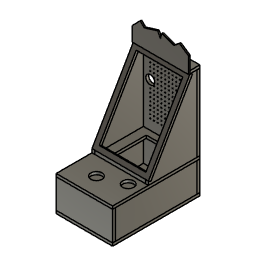
Decisioninator CAD Fusion 360 (Autodesk Fusion 360 design; units mm, degrees)
Autodesk Fusion 360 part; units mm, degrees
(part 1 of 2)
sketch "Front Bezel Sketch" plane through (0, 0, 0) normal (0, 1, 0) x (1, 0, 0)
  line L0 (-63, 93) -> (63, 93)
  line L1 (63, 93) -> (63, -93)
  line L2 (63, -93) -> (-63, -93)
  line L3 (-63, -93) -> (-63, 93)
  line L4 (-63, 93) -> (63, -93) construction
  line L5 (63, 93) -> (-63, -93) construction
  line L6 (50, 80) -> (-50, 80)
  line L7 (-50, 80) -> (-50, -80)
  line L8 (-50, -80) -> (50, -80)
  line L9 (50, -80) -> (50, 80)
  line L10 (50, 80) -> (-50, -80) construction
  line L11 (-50, 80) -> (50, -80) construction
  dimension "d3" = 126
  dimension "d4" = 186
  dimension "d5" = 100
  dimension "d6" = 160
  constraint horizontal L0
  constraint perpendicular L0 L1
  constraint parallel L0 L2
  constraint parallel L1 L3
  constraint coincident L4 origin
  constraint coincident L5 origin
  constraint horizontal L6
  constraint perpendicular L6 L7
  constraint parallel L6 L8
  constraint parallel L7 L9
  constraint coincident L10 origin
  constraint coincident L11 origin
  measures "d3" distance of L1.end L2.end
  measures "d4" distance of L0.end L1.end
  measures "d5" distance of L7.end L8.end
  measures "d6" distance of L6.end L7.end
extrude "Extrude1" add sketch "Front Bezel Sketch" along normal blind 6.35 makes body 1
sketch "Top Case Sketch" plane through (0, 6.35, 0) normal (0, 1, 0) x (-1, 0, 0)
  line L0 (-50, -80) -> (-50, 80)
  line L1 (-50, 80) -> (50, 80)
  line L2 (50, 80) -> (50, -80)
  line L3 (50, -80) -> (-50, -80)
  line L4 (63, 93) -> (-63, 93)
  line L5 (-63, 93) -> (-63, -93)
  line L6 (-63, -93) -> (63, -93)
  line L7 (63, -93) -> (63, 93)
  line L8 (-56.65, 86.65) -> (56.65, 86.65)
  line L9 (56.65, 86.65) -> (56.65, -86.65)
  line L10 (56.65, -86.65) -> (-56.65, -86.65)
  line L11 (-56.65, -86.65) -> (-56.65, 86.65)
  dimension "d9" = 6.35
  dimension "d10" = 6.35
  dimension "d11" = 6.35
  dimension "d12" = 6.35
  constraint horizontal L8
  constraint vertical L9
  constraint horizontal L10
  constraint vertical L11
  measures "d9" distance of L5 L11
  measures "d10" distance of L7 L9
  measures "d11" distance of L4 L8
  measures "d12" distance of L6 L10
move_body "Move1" bodies 1 to x (1, 0, 0) y (0, 0.866025, -0.5) z (0, 0.5, 0.866025) at (0, -42.6114, 14.8206)
sketch "Side" plane through (63, 0, 0) normal (1, 0, 0) x (0, 1, 0)
  line L0 (3.8886, 95.361) -> (-89.1114, -65.7197)
  line L1 (-89.1114, -65.7197) -> (-83.6122, -68.8947)
  line L2 (-83.6122, -68.8947) -> (9.3878, 92.186)
  line L3 (9.3878, 92.186) -> (3.8886, 95.361)
  line L4 (-83.6122, -68.8947) -> (10, -68.8947)
  line L5 (9.3878, 92.186) -> (9.3878, -70)
  constraint coincident L1.end L2.start
  constraint horizontal L4
  constraint coincident L2.end L3.start
  constraint perpendicular L4 L5
extrude "Extrude12" add sketch "Side" against normal blind 6.35 separate body contours L2 L4 L5 makes body 2
sketch "Sketch6" plane through (56.65, 0, 0) normal (-1, 0, 0) x (0, -1, 0)
  line L0 (-9.3878, -68.8947) -> (83.6122, -68.8947)
  line L1 (83.6122, -68.8947) -> (-9.3878, 92.186)
  line L2 (-9.3878, 92.186) -> (-9.3878, -68.8947)
extrude "Extrude13" add 1 faces at (60.8833, 9.3878, 38.4924) along direction (0, 1, 0) blind 10 on bodies 2 bodies 2
sketch "Sketch7" plane through (63, 0, 0) normal (1, 0, 0) x (0, 1, 0)
  line L0 (-83.6122, -68.8947) -> (19.3878, -68.8947)
  line L1 (19.3878, -68.8947) -> (19.3878, 92.186)
  line L2 (19.3878, 92.186) -> (9.3878, 92.186)
  line L3 (9.3878, 92.186) -> (-83.6122, -68.8947)
  line L4 (3.8886, 95.361) -> (9.3878, 92.186)
  line L5 (-89.1114, -65.7197) -> (3.8886, 95.361)
  line L6 (-83.6122, -68.8947) -> (9.3878, 92.186)
  line L7 (3.8886, 95.361) -> (20, 95.361)
  line L8 (19.3878, 92.186) -> (19.3878, 95.361)
  point P0 (3.8886, 95.361)
  point P1 (9.3878, 92.186)
  constraint coincident P0 L4.start
  constraint horizontal L7
  constraint coincident L1.end L2.start
  constraint coincident L7 L8.end
  constraint perpendicular L7 L8
extrude "Extrude14" add sketch "Sketch7" against normal blind 6.35 contours L2 L4 L7 L8 bodies 2
copy_body "CopyPasteBodies1" bodies 2 makes body 3
extrude "Extrude15" add 1 faces at (60.8833, -49.2788, -68.8947) along direction (0, 0, -1) blind 5 on bodies 2 bodies 2 3
sketch "Sketch8" plane through (63, 0, 0) normal (1, 0, 0) x (0, 1, 0)
  line L0 (3.8886, 95.361) -> (-89.1114, -65.7197)
  line L1 (-89.1114, -65.7197) -> (-83.6122, -68.8947)
  line L2 (-83.6122, -68.8947) -> (9.3878, 92.186)
  line L3 (9.3878, 92.186) -> (3.8886, 95.361)
  line L4 (-89.1114, -65.7197) -> (-89.1114, -73.8947)
  line L5 (-89.1114, -73.8947) -> (-83.5716, -73.8947)
  line L6 (-83.6122, -68.8947) -> (-83.6122, -73.8947)
  line L7 (19.3878, -73.8947) -> (-83.6122, -73.8947)
  constraint coincident L0.end L1.start
  constraint parallel L4 L6
  constraint collinear L5 L7
extrude "Extrude16" add sketch "Sketch8" against normal blind 6.35 contours L1 L4 L5 L6 bodies 2
copy_body "CopyPasteBodies2" bodies 2 makes body 4
move_body "Move3" bodies 4 to x (1, 0, 0) y (0, 1, 0) z (0, 0, 1) at (-110, 0, 0)
move_body "Align2" bodies 4 to x (1, 0, 0) y (0, 1, 0) z (0, 0, 1) at (-9.65, 0, 0)
sketch "Sketch9" plane through (56.65, 0, 0) normal (-1, 0, 0) x (0, -1, 0)
  line L0 (83.6122, -68.8947) -> (-9.3878, 92.186)
  line L1 (-9.3878, 92.186) -> (-3.8886, 95.361)
  line L2 (-3.8886, 95.361) -> (-19.3878, 95.361)
  line L3 (-19.3878, 95.361) -> (-19.3878, -73.8947)
  line L4 (-19.3878, -73.8947) -> (89.1114, -73.8947)
  line L5 (89.1114, -73.8947) -> (89.1114, -65.7197)
  line L6 (89.1114, -65.7197) -> (83.6122, -68.8947)
  line L7 (89.1114, -65.7197) -> (83.6122, -68.8947)
  line L8 (89.1114, -65.7197) -> (89.1114, -73.8947)
  line L9 (83.6122, -68.8947) -> (83.6122, -73.8947)
  line L10 (89.1114, -73.8947) -> (83.5716, -73.8947)
extrude "Extrude17" add sketch "Sketch9" along normal up to surface (113.3 mm away) separate body contours L4 L5 L6 L7 L8 L9 L10 makes body 5
sketch "Sketch10" plane through (0, 19.3878, 0) normal (0, 1, 0) x (-1, 0, 0)
  line L0 (-63, 95.361) -> (-63, -73.8947)
  line L1 (-63, -73.8947) -> (-56.65, -73.8947)
  line L2 (-56.65, -73.8947) -> (-56.65, 95.361)
  line L3 (-56.65, 95.361) -> (-63, 95.361)
  line L4 (63, 95.361) -> (63, -73.8947)
  line L5 (-56.65, -73.8947) -> (56.65, -73.8947)
  line L6 (63, -73.8947) -> (56.65, -73.8947)
  line L7 (-56.65, -73.8947) -> (-63, -73.8947)
  line L8 (-63, -68.8947) -> (-63, 92.186)
  line L9 (-63, 92.186) -> (-63, 95.361)
  line L10 (-63, 95.361) -> (-56.65, 95.361)
  line L11 (-63, 95.361) -> (63, 95.361)
  line L12 (-63, 95.361) -> (63, 95.361)
  line L13 (63, 95.361) -> (63, -73.8947)
  line L14 (63, -73.8947) -> (-63, -73.8947)
  line L15 (-63, -73.8947) -> (-63, 95.361)
  point P0 (63, -73.8947)
  constraint horizontal L12
  constraint vertical L13
  constraint horizontal L14
  constraint vertical L15
  constraint coincident P0 L4.end
  constraint coincident L0.start L3.end
extrude "Extrude18" add sketch "Sketch10" along normal blind 6.35 separate body makes body 6
sketch "Sketch11" plane through (0, 25.7378, 0) normal (0, 1, 0) x (-1, 0, 0)
  line L0 (-63, -73.8947) -> (63, -73.8947)
  line L1 (63, -73.8947) -> (63, 95.361)
  line L2 (63, 95.361) -> (-63, 95.361)
  line L3 (-63, 95.361) -> (-63, -73.8947)
  line L4 (-46.65, 79.011) -> (46.65, 79.011)
  line L5 (46.65, 79.011) -> (46.65, -57.5447)
  line L6 (46.65, -57.5447) -> (-46.65, -57.5447)
  line L7 (-46.65, -57.5447) -> (-46.65, 79.011)
  circle A0 centre (-41.65, 74.011) radius 1.25
  dimension "d63" = 16.35
  dimension "d64" = 16.35
  dimension "d65" = 16.35
  dimension "d66" = 16.35
  dimension "d67" = 2.5
  dimension "d68" = 5
  dimension "d69" = 5
  constraint horizontal L4
  constraint vertical L5
  constraint horizontal L6
  constraint vertical L7
  measures "d63" distance of L3 L7
  measures "d64" distance of L1 L5
  measures "d65" distance of L2 L4
  measures "d66" distance of L0 L6
  measures "d67" diameter of A0
  measures "d68" distance of L7 A0.centre
  measures "d69" distance of L4 A0.centre
extrude "Extrude19" cut sketch "Sketch11" against normal blind 6.35 contours A0 bodies 6
pattern_linear "R-Pattern4" count 16 spacing 8.3333 along (0, 0, -1) count 11 spacing 8.3 along (-1, 0, 0) of "Extrude19"
extrude "Extrude20" add 1 faces at (58.7667, 9.055, 95.361) along direction (0, 0, 1) blind 6.35 separate body on bodies 2 makes body 7
extrude "Extrude21" add 1 faces at (-60.8833, 9.055, 95.361) along direction (0, 0, 1) blind 6.35 separate body on bodies 4 makes body 8
extrude "Extrude22" add 1 faces at (-56.65, 9.055, 97.4777) along direction (1, 0, 0) up to near side of body 7 separate body on bodies 8 makes body 9
combine "Combine1" operation add target body 9 tool bodies 8
combine "Combine2" operation add target body 9 tool bodies 7
extrude "Extrude23" add 1 faces at (60.8833, -52.945, -73.8947) along direction (0, 0, -1) blind 6.35 separate body on bodies 2 makes body 10
extrude "Extrude24" add 1 faces at (60.8833, 19.3878, -76.0114) along direction (0, 1, 0) blind 6.35 on bodies 10 bodies 10
extrude "Extrude25" add 1 faces at (56.65, -12.5452, -76.0114) along direction (-1, 0, 0) blind 119.65 on bodies 10 bodies 10
extrude "Extrude26" add 1 faces at (-21, -89.1114, -78.128) along direction (0, -1, 0) blind 80 on bodies 10 bodies 10
sketch "Sketch12" plane through (0, 0, -73.8947) normal (0, 0, 1) x (-1, 0, 0)
  line L0 (-63, 169.1114) -> (-63, -25.7378)
  line L1 (-63, -25.7378) -> (63, -25.7378)
  line L2 (63, -25.7378) -> (63, 169.1114)
  line L3 (63, 169.1114) -> (-63, 169.1114)
  line L4 (36.65, -5.7378) -> (-36.65, -5.7378)
  line L5 (-36.65, -5.7378) -> (-36.65, 69.1114)
  line L6 (-36.65, 69.1114) -> (36.65, 69.1114)
  line L7 (36.65, 69.1114) -> (36.65, -5.7378)
  line L8 (56.65, -19.3878) -> (56.65, 89.1114)
  line L9 (-56.65, -19.3878) -> (-56.65, 89.1114)
  dimension "d90" = 20
  dimension "d91" = 20
  dimension "d92" = 20
  dimension "d93" = 20
  constraint horizontal L4
  constraint vertical L5
  constraint horizontal L6
  constraint vertical L7
  measures "d90" distance of L7 L8
  measures "d91" distance of L5 L9
  measures "d92" distance of L1 L4
  measures "d93" distance of L6 L8.end
extrude "Extrude27" cut sketch "Sketch12" against normal blind 6.35 contours L4 L5 L6 L7 bodies 10
extrude "Extrude28" add 1 faces at (21, 19.3878, 99.5943) along direction (0, 1, 0) blind 6.35 on bodies 9 bodies 9
sketch "Sketch13" plane through (0, 0, -80.2447) normal (0, 0, -1) x (1, 0, 0)
  line L0 (36.65, 69.1114) -> (36.65, -5.7378)
  line L1 (36.65, -5.7378) -> (-36.65, -5.7378)
  line L2 (-36.65, -5.7378) -> (-36.65, 69.1114)
  line L3 (-36.65, 69.1114) -> (36.65, 69.1114)
  line L4 (63, -25.7378) -> (63, 169.1114)
  line L5 (63, 169.1114) -> (-63, 169.1114)
  line L6 (-63, 169.1114) -> (-63, -25.7378)
  line L7 (-63, -25.7378) -> (63, -25.7378)
  line L8 (-63, 162.7614) -> (63, 162.7614)
  line L9 (-63, -19.3878) -> (63, -19.3878)
  line L10 (56.65, 162.7614) -> (56.65, -19.3878)
  line L11 (-56.65, 162.7614) -> (-56.65, -19.3878)
  dimension "d98" = 6.35
  dimension "d99" = 6.35
  dimension "d100" = 6.35
  dimension "d101" = 6.35
  constraint coincident L6 L8.start
  constraint coincident L4 L8.end
  constraint perpendicular L4 L8
  constraint coincident L6 L9.start
  constraint coincident L4 L9.end
  constraint perpendicular L4 L9
  constraint coincident L8 L10.start
  constraint coincident L9 L10.end
  constraint perpendicular L9 L10
  constraint coincident L8 L11.start
  constraint perpendicular L1 L11
  measures "d98" distance of L5 L8
  measures "d99" distance of L7 L9
  measures "d100" distance of L6 L11
  measures "d101" distance of L4 L10
extrude "Extrude29" add sketch "Sketch13" along normal blind 80 separate body contours L4 L5 L6 L8 makes body 11
extrude "Extrude30" add sketch "Sketch13" along normal blind 80 separate body contours L6 L8 L9 L11 makes body 12
extrude "Extrude31" add sketch "Sketch13" along normal blind 80 separate body contours L4 L6 L7 L9 makes body 13
extrude "Extrude32" add sketch "Sketch13" along normal blind 80 separate body contours L4 L8 L9 L10 makes body 14
extrude "Extrude33" cut 4 faces at (60.8833, -41.3286, -160.2447) (18.8833, 23.6212, -160.2447) (-58.7667, -102.045, -160.2447) (-18.8833, -166.9948, -160.2447) along direction (0, 0, 1) blind 15 on bodies 11 12 13 14 bodies 11 12 13 14
sketch "Sketch14" plane through (0, 0, -145.2447) normal (0, 0, -1) x (1, 0, 0)
  line L0 (63, -19.3878) -> (-63, -19.3878)
  line L1 (-63, -19.3878) -> (-63, -25.7378)
  line L2 (-63, -25.7378) -> (63, -25.7378)
  line L3 (63, -25.7378) -> (63, -19.3878)
  line L4 (63, -25.7378) -> (-63, -25.7378)
  line L5 (-63, -25.7378) -> (-63, 169.1114)
  line L6 (-63, 169.1114) -> (63, 169.1114)
  line L7 (63, 169.1114) -> (63, -25.7378)
  line L8 (-63, 169.1114) -> (-63, -25.7378)
  line L9 (63, 169.1114) -> (-63, 169.1114)
  constraint horizontal L4
  constraint vertical L5
  constraint horizontal L6
  constraint vertical L7
  constraint coincident L2.end L3.start
  constraint collinear L5 L8
  constraint collinear L6 L9
extrude "Extrude34" add sketch "Sketch14" along normal blind 6.35 separate body makes body 15
sketch "Sketch15" plane through (0, 25.7378, 0) normal (0, 1, 0) x (-1, 0, 0)
  circle A0 centre (41.35, -50.989) radius 1.25
  circle A1 centre (41.35, -42.6557) radius 1.25
  circle A2 centre (41.35, -34.3223) radius 1.25
  circle A3 centre (41.35, -25.989) radius 1.25
  circle A4 centre (41.35, -17.6557) radius 1.25
  circle A5 centre (41.35, -9.3223) radius 1.25
  circle A6 centre (41.35, -0.989) radius 1.25
  circle A7 centre (41.35, 7.3443) radius 1.25
  circle A8 centre (41.35, 15.6777) radius 1.25
  circle A9 centre (41.35, 24.011) radius 1.25
  circle A10 centre (41.35, 32.3443) radius 1.25
  circle A11 centre (41.35, 40.6777) radius 1.25
  circle A12 centre (41.35, 49.011) radius 1.25
  circle A13 centre (41.35, 57.3443) radius 1.25
  circle A14 centre (41.35, 65.6777) radius 1.25
  circle A15 centre (41.35, 74.011) radius 1.25
  circle A16 centre (33.05, -50.989) radius 1.25
  circle A17 centre (33.05, -42.6557) radius 1.25
  circle A18 centre (33.05, -34.3223) radius 1.25
  circle A19 centre (33.05, -25.989) radius 1.25
  circle A20 centre (33.05, -17.6557) radius 1.25
  circle A21 centre (33.05, -9.3223) radius 1.25
  circle A22 centre (33.05, -0.989) radius 1.25
  circle A23 centre (33.05, 7.3443) radius 1.25
  circle A24 centre (33.05, 15.6777) radius 1.25
  circle A25 centre (33.05, 24.011) radius 1.25
  circle A26 centre (33.05, 32.3443) radius 1.25
  circle A27 centre (33.05, 40.6777) radius 1.25
  circle A28 centre (33.05, 49.011) radius 1.25
  circle A29 centre (33.05, 57.3443) radius 1.25
  circle A30 centre (33.05, 65.6777) radius 1.25
  circle A31 centre (33.05, 74.011) radius 1.25
  circle A32 centre (24.75, -50.989) radius 1.25
  circle A33 centre (24.75, -42.6557) radius 1.25
  circle A34 centre (24.75, -34.3223) radius 1.25
  circle A35 centre (24.75, -25.989) radius 1.25
  circle A36 centre (24.75, -17.6557) radius 1.25
  circle A37 centre (24.75, -9.3223) radius 1.25
  circle A38 centre (24.75, -0.989) radius 1.25
  circle A39 centre (24.75, 7.3443) radius 1.25
  circle A40 centre (24.75, 15.6777) radius 1.25
  circle A41 centre (24.75, 24.011) radius 1.25
  circle A42 centre (24.75, 32.3443) radius 1.25
  circle A43 centre (24.75, 40.6777) radius 1.25
  circle A44 centre (24.75, 49.011) radius 1.25
  circle A45 centre (24.75, 57.3443) radius 1.25
  circle A46 centre (24.75, 65.6777) radius 1.25
  circle A47 centre (24.75, 74.011) radius 1.25
  circle A48 centre (16.45, -50.989) radius 1.25
  circle A49 centre (16.45, -42.6557) radius 1.25
  circle A50 centre (16.45, -34.3223) radius 1.25
  circle A51 centre (16.45, -25.989) radius 1.25
  circle A52 centre (16.45, -17.6557) radius 1.25
  circle A53 centre (16.45, -9.3223) radius 1.25
  circle A54 centre (16.45, -0.989) radius 1.25
  circle A55 centre (16.45, 7.3443) radius 1.25
  circle A56 centre (16.45, 15.6777) radius 1.25
  circle A57 centre (16.45, 24.011) radius 1.25
  circle A58 centre (16.45, 32.3443) radius 1.25
  circle A59 centre (16.45, 40.6777) radius 1.25
  circle A60 centre (16.45, 49.011) radius 1.25
  circle A61 centre (16.45, 57.3443) radius 1.25
  circle A62 centre (16.45, 65.6777) radius 1.25
  circle A63 centre (16.45, 74.011) radius 1.25
  circle A64 centre (8.15, -50.989) radius 1.25
  circle A65 centre (8.15, -42.6557) radius 1.25
  circle A66 centre (8.15, -34.3223) radius 1.25
  circle A67 centre (8.15, -25.989) radius 1.25
  circle A68 centre (8.15, -17.6557) radius 1.25
  circle A69 centre (8.15, -9.3223) radius 1.25
  circle A70 centre (8.15, -0.989) radius 1.25
  circle A71 centre (8.15, 7.3443) radius 1.25
  circle A72 centre (8.15, 15.6777) radius 1.25
  circle A73 centre (8.15, 24.011) radius 1.25
  circle A74 centre (8.15, 32.3443) radius 1.25
  circle A75 centre (8.15, 40.6777) radius 1.25
  circle A76 centre (8.15, 49.011) radius 1.25
  circle A77 centre (8.15, 57.3443) radius 1.25
  circle A78 centre (8.15, 65.6777) radius 1.25
  circle A79 centre (8.15, 74.011) radius 1.25
  circle A80 centre (-0.15, -50.989) radius 1.25
  circle A81 centre (-0.15, -42.6557) radius 1.25
  circle A82 centre (-0.15, -34.3223) radius 1.25
  circle A83 centre (-0.15, -25.989) radius 1.25
  circle A84 centre (-0.15, -17.6557) radius 1.25
  circle A85 centre (-0.15, -9.3223) radius 1.25
  circle A86 centre (-0.15, -0.989) radius 1.25
  circle A87 centre (-0.15, 7.3443) radius 1.25
  circle A88 centre (-0.15, 15.6777) radius 1.25
  circle A89 centre (-0.15, 24.011) radius 1.25
  circle A90 centre (-0.15, 32.3443) radius 1.25
  circle A91 centre (-0.15, 40.6777) radius 1.25
  circle A92 centre (-0.15, 49.011) radius 1.25
  circle A93 centre (-0.15, 57.3443) radius 1.25
  circle A94 centre (-0.15, 65.6777) radius 1.25
  circle A95 centre (-0.15, 74.011) radius 1.25
  circle A96 centre (-8.45, -50.989) radius 1.25
  circle A97 centre (-8.45, -42.6557) radius 1.25
  circle A98 centre (-8.45, -34.3223) radius 1.25
  circle A99 centre (-8.45, -25.989) radius 1.25
  circle A100 centre (-8.45, -17.6557) radius 1.25
  circle A101 centre (-8.45, -9.3223) radius 1.25
  circle A102 centre (-8.45, -0.989) radius 1.25
  circle A103 centre (-8.45, 7.3443) radius 1.25
  circle A104 centre (-8.45, 15.6777) radius 1.25
  circle A105 centre (-8.45, 24.011) radius 1.25
  circle A106 centre (-8.45, 32.3443) radius 1.25
  circle A107 centre (-8.45, 40.6777) radius 1.25
  circle A108 centre (-8.45, 49.011) radius 1.25
  circle A109 centre (-8.45, 57.3443) radius 1.25
  circle A110 centre (-8.45, 65.6777) radius 1.25
  circle A111 centre (-8.45, 74.011) radius 1.25
  circle A112 centre (-16.75, -50.989) radius 1.25
  circle A113 centre (-16.75, -42.6557) radius 1.25
  circle A114 centre (-16.75, -34.3223) radius 1.25
  circle A115 centre (-16.75, -25.989) radius 1.25
  circle A116 centre (-16.75, -17.6557) radius 1.25
  circle A117 centre (-16.75, -9.3223) radius 1.25
  circle A118 centre (-16.75, -0.989) radius 1.25
  circle A119 centre (-16.75, 7.3443) radius 1.25
  circle A120 centre (-16.75, 15.6777) radius 1.25
  circle A121 centre (-16.75, 24.011) radius 1.25
  circle A122 centre (-16.75, 32.3443) radius 1.25
  circle A123 centre (-16.75, 40.6777) radius 1.25
  circle A124 centre (-16.75, 49.011) radius 1.25
  circle A125 centre (-16.75, 57.3443) radius 1.25
  circle A126 centre (-16.75, 65.6777) radius 1.25
  circle A127 centre (-16.75, 74.011) radius 1.25
  circle A128 centre (-25.05, -50.989) radius 1.25
  circle A129 centre (-25.05, -42.6557) radius 1.25
  circle A130 centre (-25.05, -34.3223) radius 1.25
  circle A131 centre (-25.05, -25.989) radius 1.25
  circle A132 centre (-25.05, -17.6557) radius 1.25
  circle A133 centre (-25.05, -9.3223) radius 1.25
  circle A134 centre (-25.05, -0.989) radius 1.25
  circle A135 centre (-25.05, 7.3443) radius 1.25
  circle A136 centre (-25.05, 15.6777) radius 1.25
  circle A137 centre (-25.05, 24.011) radius 1.25
  circle A138 centre (-25.05, 32.3443) radius 1.25
  circle A139 centre (-25.05, 40.6777) radius 1.25
  circle A140 centre (-25.05, 49.011) radius 1.25
  circle A141 centre (-25.05, 57.3443) radius 1.25
  circle A142 centre (-25.05, 65.6777) radius 1.25
  circle A143 centre (-25.05, 74.011) radius 1.25
  circle A144 centre (-33.35, -50.989) radius 1.25
  circle A145 centre (-33.35, -42.6557) radius 1.25
  circle A146 centre (-33.35, -34.3223) radius 1.25
  circle A147 centre (-33.35, -25.989) radius 1.25
  circle A148 centre (-33.35, -17.6557) radius 1.25
  circle A149 centre (-33.35, -9.3223) radius 1.25
  circle A150 centre (-33.35, -0.989) radius 1.25
  circle A151 centre (-33.35, 7.3443) radius 1.25
  circle A152 centre (-33.35, 15.6777) radius 1.25
  circle A153 centre (-33.35, 24.011) radius 1.25
  circle A154 centre (-33.35, 32.3443) radius 1.25
  circle A155 centre (-33.35, 40.6777) radius 1.25
  circle A156 centre (-33.35, 49.011) radius 1.25
  circle A157 centre (-33.35, 57.3443) radius 1.25
  circle A158 centre (-33.35, 65.6777) radius 1.25
  circle A159 centre (-33.35, 74.011) radius 1.25
  circle A160 centre (-41.65, -50.989) radius 1.25
  circle A161 centre (-41.65, -42.6557) radius 1.25
  circle A162 centre (-41.65, -34.3223) radius 1.25
  circle A163 centre (-41.65, -25.989) radius 1.25
  circle A164 centre (-41.65, -17.6557) radius 1.25
  circle A165 centre (-41.65, -9.3223) radius 1.25
  circle A166 centre (-41.65, -0.989) radius 1.25
  circle A167 centre (-41.65, 7.3443) radius 1.25
  circle A168 centre (-41.65, 15.6777) radius 1.25
  circle A169 centre (-41.65, 24.011) radius 1.25
  circle A170 centre (-41.65, 32.3443) radius 1.25
  circle A171 centre (-41.65, 40.6777) radius 1.25
  circle A172 centre (-41.65, 49.011) radius 1.25
  circle A173 centre (-41.65, 57.3443) radius 1.25
  circle A174 centre (-41.65, 65.6777) radius 1.25
  circle A175 centre (-41.65, 74.011) radius 1.25
  line L0 (-63, -73.8947) -> (63, -73.8947)
  line L1 (63, -73.8947) -> (63, 95.361)
  line L2 (63, 95.361) -> (-63, 95.361)
  line L3 (-63, 95.361) -> (-63, -73.8947)
  circle A176 centre (41.35, 24.011) radius 10
  dimension "d114" = 20
  constraint coincident A9.centre A176.centre
  measures "d114" diameter of A176
extrude "Extrude35" cut sketch "Sketch15" against normal blind 20 contours A176 bodies 6
sketch "Sketch16" plane through (0, 0, -151.5947) normal (0, 0, -1) x (1, 0, 0)
  line L0 (63, -25.7378) -> (63, 169.1114)
  line L1 (63, 169.1114) -> (-63, 169.1114)
  line L2 (-63, 169.1114) -> (-63, -25.7378)
  line L3 (-63, -25.7378) -> (63, -25.7378)
  circle A0 centre (0, 0) radius 10
  dimension "d117" = 20
  constraint coincident A0.centre origin
  measures "d117" diameter of A0
extrude "Extrude36" cut sketch "Sketch16" against normal blind 50 contours A0 bodies 15
sketch "Sketch17" plane through (0, 0, -73.8947) normal (0, 0, 1) x (-1, 0, 0)
  line L0 (-36.65, -5.7378) -> (-36.65, 69.1114)
  line L1 (-36.65, 69.1114) -> (36.65, 69.1114)
  line L2 (36.65, 69.1114) -> (36.65, -5.7378)
  line L3 (36.65, -5.7378) -> (-36.65, -5.7378)
  line L4 (-63, 169.1114) -> (-63, -25.7378)
  line L5 (-63, -25.7378) -> (63, -25.7378)
  line L6 (63, -25.7378) -> (63, 169.1114)
  line L7 (63, 169.1114) -> (-63, 169.1114)
  circle A0 centre (13, 129.1114) radius 12.5
  circle A1 centre (13, 129.1114) radius 30.25
  circle A2 centre (-38, 109.1114) radius 16.5
  line L8 (-56.65, 89.1114) -> (56.65, 89.1114)
  circle A3 centre (-38, 109.1114) radius 12.5
  dimension "d120" = 25
  dimension "d121" = 50
  dimension "d122" = 40
  dimension "d124" = 60.5
  dimension "d125" = 33
  dimension "d126" = 20
  dimension "d127" = 25
  dimension "d128" = 25
  constraint concentric A0 A1
  constraint concentric A2 A3
  measures "d120" diameter of A0
  measures "d121" distance of L6 A0.centre
  measures "d122" distance of L7 A0.centre
  measures "d124" diameter of A1
  measures "d125" diameter of A2
  measures "d126" distance of A2.centre L8
  measures "d127" distance of L4 A2.centre
  measures "d128" diameter of A3
extrude "Extrude37" cut sketch "Sketch17" against normal blind 7.62 contours A0 bodies 10
extrude "Extrude38" cut sketch "Sketch17" against normal blind 7.62 contours A3 bodies 10
sketch "Sketch18" plane through (0, 0, 101.711) normal (0, 0, 1) x (-1, 0, 0)
  line L0 (63, -25.7378) -> (63, -3.8886)
  line L1 (63, -3.8886) -> (-63, -3.8886)
  line L2 (-63, -3.8886) -> (-63, -25.7378)
  line L3 (-63, -25.7378) -> (63, -25.7378)
  line L4 (63, -3.8886) -> (-63, -3.8886)
  line L5 (-63, -3.8886) -> (-63, -7.0636)
  line L6 (-63, -7.0636) -> (63, -7.0636)
  line L7 (63, -7.0636) -> (63, -3.8886)
  dimension "d133" = 3.175
  constraint horizontal L4
  constraint vertical L5
  constraint horizontal L6
  constraint vertical L7
  constraint coincident L2 L5.end
  constraint coincident L0.end L1.start
  measures "d133" distance of L4 L6
extrude "Extrude39" add sketch "Sketch18" along normal blind 50 separate body contours L0 L1 L2 L4 L5 L6 L7 makes body 16
sketch "Sketch19" plane through (0, 3.8886, 0) normal (0, -1, 0) x (1, 0, 0)
  line L0 (-63, 101.711) -> (63, 101.711)
  line L1 (63, 101.711) -> (63, 151.711)
  line L2 (63, 151.711) -> (-63, 151.711)
  line L3 (-63, 151.711) -> (-63, 101.711)
  line L4 (-63, 133.5614) -> (-45.2775, 151.711)
  line L5 (-45.2775, 151.711) -> (-35.984, 142.6362)
  line L6 (-35.984, 142.6362) -> (-6.8129, 151.711)
  line L7 (-5.8194, 151.711) -> (0, 140)
  line L8 (0, 140) -> (3.4065, 151.711)
  line L9 (3.4065, 151.711) -> (30.0903, 141.6517)
  line L10 (30.0903, 141.6517) -> (42.5807, 151.711)
  line L11 (42.5807, 151.711) -> (63, 137.9614)
  constraint coincident L3 L4.start
  constraint coincident L2 L4.end
  constraint perpendicular L4 L5
  constraint coincident L2 L6.end
  constraint coincident L2 L7.start
  constraint coincident L2 L8.end
  constraint coincident L2 L10.end
  constraint coincident L1 L11.end
extrude "Extrude40" cut sketch "Sketch19" against normal blind 85 contours L2 L3 L4 | L1 L2 L11 | L2 L5 L6 | L2 L9 L10 | L2 L7 L8 bodies 16
move_body "Align3" bodies 16 to x (1, 0, 0) y (0, 1, 0) z (0, 0, 1) at (0, -3.175, -6.35)
copy_body "CopyPasteBodies3" bodies 1 makes body 17
sketch "Sketch21" plane through (63, 0, 0) normal (1, 0, 0) x (0, 1, 0)
  line L0 (19.3878, -73.8947) -> (19.3878, 95.361)
  line L1 (19.3878, 95.361) -> (3.8886, 95.361)
  line L2 (3.8886, 95.361) -> (9.3878, 92.186)
  line L3 (9.3878, 92.186) -> (-83.6122, -68.8947)
  line L4 (-83.6122, -68.8947) -> (-89.1114, -65.7197)
  line L5 (-89.1114, -65.7197) -> (-89.1114, -73.8947)
  line L6 (-89.1114, -73.8947) -> (19.3878, -73.8947)
  line L7 (3.8886, 95.361) -> (-89.1114, -65.7197)
  line L8 (3.8886, 95.361) -> (3.8886, 101.711)
  line L9 (3.8886, 101.711) -> (25.7378, 101.711)
  line L10 (25.7378, 101.711) -> (25.7378, 95.361)
  line L11 (25.7378, 95.361) -> (25.7378, -73.8947)
  line L12 (25.7378, -73.8947) -> (25.7378, -80.2447)
  line L13 (25.7378, -80.2447) -> (25.7378, -145.2447)
  line L14 (25.7378, -145.2447) -> (25.7378, -151.5947)
  line L15 (25.7378, -151.5947) -> (-169.1114, -151.5947)
  line L16 (-169.1114, -145.2447) -> (-169.1114, -151.5947)
  line L17 (-169.1114, -80.2447) -> (-169.1114, -145.2447)
  line L18 (-169.1114, -80.2447) -> (-169.1114, -73.8947)
  line L19 (-89.1114, -65.7197) -> (-89.1114, -73.8947)
  line L20 (-169.1114, -73.8947) -> (-89.1114, -73.8947)
  constraint coincident L18.end L20.start
  constraint coincident L5.end L6.start
sketch "Sketch22" plane through (0, 0, -73.8947) normal (0, 0, 1) x (-1, 0, 0)
  circle A0 centre (-38, 109.1114) radius 12.5
  circle A1 centre (13, 129.1114) radius 12.5
  line L0 (-36.65, -5.7378) -> (-36.65, 69.1114)
  line L1 (-36.65, 69.1114) -> (36.65, 69.1114)
  line L2 (36.65, 69.1114) -> (36.65, -5.7378)
  line L3 (36.65, -5.7378) -> (-36.65, -5.7378)
  line L4 (-63, 169.1114) -> (-63, -25.7378)
  line L5 (-63, -25.7378) -> (63, -25.7378)
  line L6 (63, -25.7378) -> (63, 169.1114)
  line L7 (63, 169.1114) -> (-63, 169.1114)
  line L8 (63, 89.1114) -> (-63, 89.1114)
  line L9 (-63, 169.1114) -> (63, 169.1114)
  circle A2 centre (13, 129.1114) radius 12.5
  circle A3 centre (-38, 109.1114) radius 12.5
  line L10 (63, 89.1114) -> (63, 169.1114)
  line L11 (-63, 89.1114) -> (-63, 169.1114)
  constraint coincident L8.start L10.start
  constraint coincident L6.end L7.start
  constraint coincident L8.end L11.start
  constraint coincident L4.start L7.end
copy_body "CopyPasteBodies4" bodies 16 makes body 18
move_body "Move5" bodies 18 to x (1, 0, 0) y (0, 1, 0) z (0, 0, 1) at (230, 0, 0)
move_body "Align5" bodies 18 to x (1, 0, 0) y (0, 0, 1) z (0, -1, 0) at (0, 99.2496, -3.8886)
copy_body "CopyPasteBodies5" bodies 9 makes body 19
move_body "Move6" bodies 19 to x (1, 0, 0) y (0, 1, 0) z (0, 0, 1) at (600, 0, 0)
move_body "Align6" bodies 19 to x (1, 0, 0) y (0, -1, 0) z (0, 0, -1) at (0, 29.6264, 95.361)
move_body "Move7" bodies 19 to x (1, 0, 0) y (0, 1, 0) z (0, 0, 1) at (-370, 10, 0)
copy_body "CopyPasteBodies6" bodies 6 makes body 20
move_body "Move8" bodies 20 to x (1, 0, 0) y (0, 1, 0) z (0, 0, 1) at (410, 0, 0)
move_body "Align7" bodies 20 to x (1, 0, 0) y (0, 0, 1) z (0, -1, 0) at (0, 36.471, -25.7378)
move_body "Move9" bodies 20 to x (1, 0, 0) y (0, 1, 0) z (0, 0, 1) at (-40, -70, 0)
copy_body "CopyPasteBodies7" bodies 2 makes body 21
move_body "Move10" bodies 21 to x (1, 0, 0) y (0, 1, 0) z (0, 0, 1) at (440, 0, 0)
move_body "Align8" bodies 21 to x (0, 0, -1) y (0, 1, 0) z (1, 0, 0) at (485.0044, 0, 496.65)
move_body "Move11" bodies 21 to x (0, 1, 0) y (-1, 0, 0) z (0, 0, 1) at (465.1253, -536.3497, 0)
copy_body "CopyPasteBodies8" bodies 4 makes body 22
move_body "Move12" bodies 22 to x (1, 0, 0) y (0, 1, 0) z (0, 0, 1) at (760, 0, 0)
move_body "Align9" bodies 22 to x (0, 0, -1) y (0, 1, 0) z (1, 0, 0) at (685.3544, 0, 697)
move_body "Move13" bodies 22 to x (0, -1, 0) y (1, 0, 0) z (0, 0, 1) at (561.5285, 655.7115, 0)
move_body "Align10" bodies 22 to x (1, 0, 0) y (0, -1, 0) z (0, 0, -1) at (0, -82.5771, -6.35)
move_body "Move14" bodies 22 to x (-0.996195, -0.087156, 0) y (0.087156, -0.996195, 0) z (0, 0, 1) at (1029.922, -13.5464, -320)
move_body "Align11" bodies 22 to x (1, 0, 0) y (0, -1, 0) z (0, 0, -1) at (0, -36.2417, -326.35)
move_body "Move15" bodies 22 to x (0.996195, 0.087156, 0) y (-0.087156, 0.996195, 0) z (0, 0, 1) at (3.0201, -42.5908, 0)
move_body "Move16" bodies 22 to x (-1, 0, 0) y (0, -1, 0) z (0, 0, 1) at (1027.4435, -58.1734, 0)
copy_body "CopyPasteBodies9" bodies 17 makes body 23
move_body "Move17" bodies 23 to x (1, 0, 0) y (0, 1, 0) z (0, 0, 1) at (230, 0, 0)
move_body "Align12" bodies 23 to x (1, 0, 0) y (0, -0.5, 0.866025) z (0, -0.866025, -0.5) at (0, -45.5828, 37.9629)
move_body "Move18" bodies 23 to x (1, 0, 0) y (0, 1, 0) z (0, 0, 1) at (0, -10, 0)
move_body "Move19" bodies 18 to x (1, 0, 0) y (0, 1, 0) z (0, 0, 1) at (0, -200, 0)
move_body "Move20" bodies 19 to x (0, -1, 0) y (1, 0, 0) z (0, 0, 1) at (174.2622, 185.7378, 0)
move_body "Move21" bodies 18 to x (0, 1, 0) y (-1, 0, 0) z (0, 0, 1) at (28.6169, -270.8398, 0)
copy_body "CopyPasteBodies10" bodies 10 makes body 24
move_body "Move22" bodies 24 to x (1, 0, 0) y (0, 1, 0) z (0, 0, 1) at (190, -130, 0)
move_body "Align13" bodies 24 to x (1, 0, 0) y (0, -1, 0) z (0, 0, -1) at (0, -241.2243, -80.2447)
move_body "Move23" bodies 24 to x (1, 0, 0) y (0, 1, 0) z (0, 0, 1) at (40, -210, 0)
copy_body "CopyPasteBodies11" bodies 15 makes body 25
move_body "Move24" bodies 25 to x (1, 0, 0) y (0, 1, 0) z (0, 0, 1) at (290, 0, 0)
move_body "Align14" bodies 25 to x (1, 0, 0) y (0, -1, 0) z (0, 0, -1) at (0, -143.3736, -151.5947)
move_body "Move25" bodies 25 to x (1, 0, 0) y (0, 1, 0) z (0, 0, 1) at (80, -170, 0)
copy_body "CopyPasteBodies12" bodies 11 makes body 26
move_body "Move26" bodies 26 to x (1, 0, 0) y (0, 1, 0) z (0, 0, 1) at (500, 0, 0)
move_body "Align15" bodies 26 to x (1, 0, 0) y (0, 0, 1) z (0, -1, 0) at (0, -243.0061, 162.7614)
move_body "Move27" bodies 26 to x (1, 0, 0) y (0, 1, 0) z (0, 0, 1) at (10, -40, 0)
copy_body "CopyPasteBodies13" bodies 13 makes body 27
move_body "Move28" bodies 27 to x (1, 0, 0) y (0, 1, 0) z (0, 0, 1) at (520, 0, 0)
move_body "Align16" bodies 27 to x (1, 0, 0) y (0, 0, 1) z (0, -1, 0) at (0, -87.0069, -25.7378)
move_body "Move29" bodies 27 to x (1, 0, 0) y (0, 1, 0) z (0, 0, 1) at (-10, -280, 0)
copy_body "CopyPasteBodies14" bodies 14 makes body 28
move_body "Move30" bodies 28 to x (1, 0, 0) y (0, 1, 0) z (0, 0, 1) at (580, 0, 0)
move_body "Align17" bodies 28 to x (0, 0, -1) y (0, 1, 0) z (1, 0, 0) at (716.8947, 0, 636.65)
move_body "Move31" bodies 28 to x (0, -1, 0) y (1, 0, 0) z (0, 0, 1) at (331.8374, 217.3717, 0)
copy_body "CopyPasteBodies15" bodies 28 makes body 29
move_body "Move32" bodies 29 to x (1, 0, 0) y (0, 1, 0) z (0, 0, 1) at (190, 0, 0)
move_body "Move33" bodies 26 27 to x (1, 0, 0) y (0, 1, 0) z (0, 0, 1) at (0, -20, 0)
move_body "Move34" bodies 29 to x (1, 0, 0) y (0, 1, 0) z (0, 0, 1) at (30, 0, 0)
sketch "Cuts" plane through (0, 0, 0) normal (0, 0, 1) x (-1, 0, 0)
  circle A0 centre (-370, 313.3736) radius 10
  line L0 (-433, 339.1114) -> (-433, 144.2622)
  line L1 (-433, 144.2622) -> (-307, 144.2622)
  line L2 (-307, 144.2622) -> (-307, 339.1114)
  line L3 (-307, 339.1114) -> (-433, 339.1114)
  line L4 (-468.8597, -35.9167) -> (-474.359, -39.0917)
  line L5 (-468.8597, -35.9167) -> (-468.8597, -44.0917)
  line L6 (-577.359, -44.0917) -> (-468.8597, -44.0917)
  line L7 (-561.8597, 125.1641) -> (-577.359, 125.1641)
  line L8 (-561.8597, 125.1641) -> (-567.359, 121.9891)
  line L9 (-577.359, -44.0917) -> (-577.359, 125.1641)
  line L10 (-474.359, -39.0917) -> (-567.359, 121.9891)
  line L11 (-554.2368, 117.065) -> (-548.7375, 120.24)
  line L12 (-554.2368, 117.065) -> (-554.2368, 125.24)
  line L13 (-445.7375, 125.24) -> (-554.2368, 125.24)
  line L14 (-461.2368, -44.0157) -> (-445.7375, -44.0157)
  line L15 (-461.2368, -44.0157) -> (-455.7375, -40.8407)
  line L16 (-445.7375, 125.24) -> (-445.7375, -44.0157)
  line L17 (-548.7375, 120.24) -> (-455.7375, -40.8407)
  circle A1 centre (-328.65, 57.54) radius 10
  circle A2 centre (-411.65, 107.54) radius 1.25
  line L18 (-433, -40.3657) -> (-433, 128.89)
  line L19 (-433, 128.89) -> (-307, 128.89)
  line L20 (-307, 128.89) -> (-307, -40.3657)
  line L21 (-307, -40.3657) -> (-433, -40.3657)
  circle A3 centre (-328.65, -17.46) radius 1.25
  circle A4 centre (-328.65, -9.1266) radius 1.25
  circle A5 centre (-328.65, -0.7933) radius 1.25
  circle A6 centre (-328.65, 7.54) radius 1.25
  circle A7 centre (-328.65, 15.8734) radius 1.25
  circle A8 centre (-328.65, 24.2067) radius 1.25
  circle A9 centre (-328.65, 32.54) radius 1.25
  circle A10 centre (-328.65, 40.8734) radius 1.25
  circle A11 centre (-328.65, 74.2067) radius 1.25
  circle A12 centre (-328.65, 82.54) radius 1.25
  circle A13 centre (-328.65, 90.8734) radius 1.25
  circle A14 centre (-328.65, 99.2067) radius 1.25
  circle A15 centre (-328.65, 107.54) radius 1.25
  circle A16 centre (-336.95, -17.46) radius 1.25
  circle A17 centre (-336.95, -9.1266) radius 1.25
  circle A18 centre (-336.95, -0.7933) radius 1.25
  circle A19 centre (-336.95, 7.54) radius 1.25
  circle A20 centre (-336.95, 15.8734) radius 1.25
  circle A21 centre (-336.95, 24.2067) radius 1.25
  circle A22 centre (-336.95, 32.54) radius 1.25
  circle A23 centre (-336.95, 40.8734) radius 1.25
  circle A24 centre (-336.95, 49.2067) radius 1.25
  circle A25 centre (-336.95, 65.8734) radius 1.25
  circle A26 centre (-336.95, 74.2067) radius 1.25
  circle A27 centre (-336.95, 82.54) radius 1.25
  circle A28 centre (-336.95, 90.8734) radius 1.25
  circle A29 centre (-336.95, 99.2067) radius 1.25
  circle A30 centre (-336.95, 107.54) radius 1.25
  circle A31 centre (-345.25, -17.46) radius 1.25
  circle A32 centre (-345.25, -9.1266) radius 1.25
  circle A33 centre (-345.25, -0.7933) radius 1.25
  circle A34 centre (-345.25, 7.54) radius 1.25
  circle A35 centre (-345.25, 15.8734) radius 1.25
  circle A36 centre (-345.25, 24.2067) radius 1.25
  circle A37 centre (-345.25, 32.54) radius 1.25
  circle A38 centre (-345.25, 40.8734) radius 1.25
  circle A39 centre (-345.25, 49.2067) radius 1.25
  circle A40 centre (-345.25, 57.54) radius 1.25
  circle A41 centre (-345.25, 65.8734) radius 1.25
  circle A42 centre (-345.25, 74.2067) radius 1.25
  circle A43 centre (-345.25, 82.54) radius 1.25
  circle A44 centre (-345.25, 90.8734) radius 1.25
  circle A45 centre (-345.25, 99.2067) radius 1.25
  circle A46 centre (-345.25, 107.54) radius 1.25
  circle A47 centre (-353.55, -17.46) radius 1.25
  circle A48 centre (-353.55, -9.1266) radius 1.25
  circle A49 centre (-353.55, -0.7933) radius 1.25
  circle A50 centre (-353.55, 7.54) radius 1.25
  circle A51 centre (-353.55, 15.8734) radius 1.25
  circle A52 centre (-353.55, 24.2067) radius 1.25
  circle A53 centre (-353.55, 32.54) radius 1.25
  circle A54 centre (-353.55, 40.8734) radius 1.25
  circle A55 centre (-353.55, 49.2067) radius 1.25
  circle A56 centre (-353.55, 57.54) radius 1.25
  circle A57 centre (-353.55, 65.8734) radius 1.25
  circle A58 centre (-353.55, 74.2067) radius 1.25
  circle A59 centre (-353.55, 82.54) radius 1.25
  circle A60 centre (-353.55, 90.8734) radius 1.25
  circle A61 centre (-353.55, 99.2067) radius 1.25
  circle A62 centre (-353.55, 107.54) radius 1.25
  circle A63 centre (-361.85, -17.46) radius 1.25
  circle A64 centre (-361.85, -9.1266) radius 1.25
  circle A65 centre (-361.85, -0.7933) radius 1.25
  circle A66 centre (-361.85, 7.54) radius 1.25
  circle A67 centre (-361.85, 15.8734) radius 1.25
  circle A68 centre (-361.85, 24.2067) radius 1.25
  circle A69 centre (-361.85, 32.54) radius 1.25
  circle A70 centre (-361.85, 40.8734) radius 1.25
  circle A71 centre (-361.85, 49.2067) radius 1.25
  circle A72 centre (-361.85, 57.54) radius 1.25
  circle A73 centre (-361.85, 65.8734) radius 1.25
  circle A74 centre (-361.85, 74.2067) radius 1.25
  circle A75 centre (-361.85, 82.54) radius 1.25
  circle A76 centre (-361.85, 90.8734) radius 1.25
  circle A77 centre (-361.85, 99.2067) radius 1.25
  circle A78 centre (-361.85, 107.54) radius 1.25
  circle A79 centre (-370.15, -17.46) radius 1.25
  circle A80 centre (-370.15, -9.1266) radius 1.25
  circle A81 centre (-370.15, -0.7933) radius 1.25
  circle A82 centre (-370.15, 7.54) radius 1.25
  circle A83 centre (-370.15, 15.8734) radius 1.25
  circle A84 centre (-370.15, 24.2067) radius 1.25
  circle A85 centre (-370.15, 32.54) radius 1.25
  circle A86 centre (-370.15, 40.8734) radius 1.25
  circle A87 centre (-370.15, 49.2067) radius 1.25
  circle A88 centre (-370.15, 57.54) radius 1.25
  circle A89 centre (-370.15, 65.8734) radius 1.25
  circle A90 centre (-370.15, 74.2067) radius 1.25
  circle A91 centre (-370.15, 82.54) radius 1.25
  circle A92 centre (-370.15, 90.8734) radius 1.25
  circle A93 centre (-370.15, 99.2067) radius 1.25
  circle A94 centre (-370.15, 107.54) radius 1.25
  circle A95 centre (-378.45, -17.46) radius 1.25
  circle A96 centre (-378.45, -9.1266) radius 1.25
  circle A97 centre (-378.45, -0.7933) radius 1.25
  circle A98 centre (-378.45, 7.54) radius 1.25
  circle A99 centre (-378.45, 15.8734) radius 1.25
  circle A100 centre (-378.45, 24.2067) radius 1.25
  circle A101 centre (-378.45, 32.54) radius 1.25
  circle A102 centre (-378.45, 40.8734) radius 1.25
  circle A103 centre (-378.45, 49.2067) radius 1.25
  circle A104 centre (-378.45, 57.54) radius 1.25
  circle A105 centre (-378.45, 65.8734) radius 1.25
  circle A106 centre (-378.45, 74.2067) radius 1.25
  circle A107 centre (-378.45, 82.54) radius 1.25
  circle A108 centre (-378.45, 90.8734) radius 1.25
  circle A109 centre (-378.45, 99.2067) radius 1.25
  circle A110 centre (-378.45, 107.54) radius 1.25
  circle A111 centre (-386.75, -17.46) radius 1.25
  circle A112 centre (-386.75, -9.1266) radius 1.25
  circle A113 centre (-386.75, -0.7933) radius 1.25
  circle A114 centre (-386.75, 7.54) radius 1.25
  circle A115 centre (-386.75, 15.8734) radius 1.25
  circle A116 centre (-386.75, 24.2067) radius 1.25
  circle A117 centre (-386.75, 32.54) radius 1.25
  circle A118 centre (-386.75, 40.8734) radius 1.25
  circle A119 centre (-386.75, 49.2067) radius 1.25
  circle A120 centre (-386.75, 57.54) radius 1.25
  circle A121 centre (-386.75, 65.8734) radius 1.25
  circle A122 centre (-386.75, 74.2067) radius 1.25
  circle A123 centre (-386.75, 82.54) radius 1.25
  circle A124 centre (-386.75, 90.8734) radius 1.25
  circle A125 centre (-386.75, 99.2067) radius 1.25
  circle A126 centre (-386.75, 107.54) radius 1.25
  circle A127 centre (-395.05, -17.46) radius 1.25
  circle A128 centre (-395.05, -9.1266) radius 1.25
  circle A129 centre (-395.05, -0.7933) radius 1.25
  circle A130 centre (-395.05, 7.54) radius 1.25
  circle A131 centre (-395.05, 15.8734) radius 1.25
  circle A132 centre (-395.05, 24.2067) radius 1.25
  circle A133 centre (-395.05, 32.54) radius 1.25
  circle A134 centre (-395.05, 40.8734) radius 1.25
  circle A135 centre (-395.05, 49.2067) radius 1.25
  circle A136 centre (-395.05, 57.54) radius 1.25
  circle A137 centre (-395.05, 65.8734) radius 1.25
  circle A138 centre (-395.05, 74.2067) radius 1.25
  circle A139 centre (-395.05, 82.54) radius 1.25
  circle A140 centre (-395.05, 90.8734) radius 1.25
  circle A141 centre (-395.05, 99.2067) radius 1.25
  circle A142 centre (-395.05, 107.54) radius 1.25
  circle A143 centre (-403.35, -17.46) radius 1.25
  circle A144 centre (-403.35, -9.1266) radius 1.25
  circle A145 centre (-403.35, -0.7933) radius 1.25
  circle A146 centre (-403.35, 7.54) radius 1.25
  circle A147 centre (-403.35, 15.8734) radius 1.25
  circle A148 centre (-403.35, 24.2067) radius 1.25
  circle A149 centre (-403.35, 32.54) radius 1.25
  circle A150 centre (-403.35, 40.8734) radius 1.25
  circle A151 centre (-403.35, 49.2067) radius 1.25
  circle A152 centre (-403.35, 57.54) radius 1.25
  circle A153 centre (-403.35, 65.8734) radius 1.25
  circle A154 centre (-403.35, 74.2067) radius 1.25
  circle A155 centre (-403.35, 82.54) radius 1.25
  circle A156 centre (-403.35, 90.8734) radius 1.25
  circle A157 centre (-403.35, 99.2067) radius 1.25
  circle A158 centre (-403.35, 107.54) radius 1.25
  circle A159 centre (-411.65, -17.46) radius 1.25
  circle A160 centre (-411.65, -9.1266) radius 1.25
  circle A161 centre (-411.65, -0.7933) radius 1.25
  circle A162 centre (-411.65, 7.54) radius 1.25
  circle A163 centre (-411.65, 15.8734) radius 1.25
  circle A164 centre (-411.65, 24.2067) radius 1.25
  circle A165 centre (-411.65, 32.54) radius 1.25
  circle A166 centre (-411.65, 40.8734) radius 1.25
  circle A167 centre (-411.65, 49.2067) radius 1.25
  circle A168 centre (-411.65, 57.54) radius 1.25
  circle A169 centre (-411.65, 65.8734) radius 1.25
  circle A170 centre (-411.65, 74.2067) radius 1.25
  circle A171 centre (-411.65, 82.54) radius 1.25
  circle A172 centre (-411.65, 90.8734) radius 1.25
  circle A173 centre (-411.65, 99.2067) radius 1.25
  line L22 (-274.7284, 47.6527) -> (-265.6535, 76.8237)
  line L23 (-265.6535, 76.8237) -> (-274.7284, 86.1172)
  line L24 (-274.7284, 86.1172) -> (-256.5787, 103.8398)
  line L25 (-263.0173, 40.8398) -> (-274.7284, 46.6591)
  line L26 (-274.7284, 37.4333) -> (-263.0173, 40.8398)
  line L27 (-264.6691, 10.7494) -> (-274.7284, 37.4333)
  line L28 (-274.7284, -1.7409) -> (-264.6691, 10.7494)
  line L29 (-260.9787, -22.1602) -> (-274.7284, -1.7409)
  line L30 (-274.7284, 47.6527) -> (-274.7284, 46.6591)
  line L31 (-224.7284, -22.1602) -> (-260.9787, -22.1602)
  line L32 (-224.7284, 103.8398) -> (-256.5787, 103.8398)
  line L33 (-224.7284, 103.8398) -> (-224.7284, -22.1602)
  line L34 (-188.1507, -18.7378) -> (-188.1507, 107.2622)
  line L35 (-210, 107.2622) -> (-188.1507, 107.2622)
  line L36 (-210, -18.7378) -> (-188.1507, -18.7378)
  line L37 (-210, -18.7378) -> (-210, 107.2622)
  line L38 (-180, -32.8878) -> (-280, -32.8878)
  line L39 (-180, 127.1122) -> (-180, -32.8878)
  line L40 (-280, 127.1122) -> (-180, 127.1122)
  line L41 (-280, -32.8878) -> (-280, 127.1122)
  line L42 (-167, 140.1122) -> (-167, -45.8878)
  line L43 (-167, -45.8878) -> (-293, -45.8878)
  line L44 (-293, -45.8878) -> (-293, 140.1122)
  line L45 (-293, 140.1122) -> (-167, 140.1122)
  circle A174 centre (-268, 212.1129) radius 12.5
  circle A175 centre (-217, 192.1129) radius 12.5
  line L46 (-266.65, 326.9622) -> (-266.65, 252.1129)
  line L47 (-193.35, 326.9622) -> (-266.65, 326.9622)
  line L48 (-193.35, 252.1129) -> (-193.35, 326.9622)
  line L49 (-266.65, 252.1129) -> (-193.35, 252.1129)
  line L50 (-293, 152.1129) -> (-167, 152.1129)
  line L51 (-167, 346.9622) -> (-167, 152.1129)
  line L52 (-293, 346.9622) -> (-167, 346.9622)
  line L53 (-293, 346.9622) -> (-293, 152.1129)
  circle A176 centre (-370, 313.3736) radius 10
  line L54 (-433, 339.1114) -> (-307, 339.1114)
  line L55 (-307, 144.2622) -> (-307, 339.1114)
  line L56 (-433, 144.2622) -> (-307, 144.2622)
  line L57 (-433, 144.2622) -> (-433, 339.1114)
  line L58 (-447, 157.7614) -> (-573, 157.7614)
  line L59 (-447, 222.7614) -> (-447, 157.7614)
  line L60 (-573, 222.7614) -> (-573, 157.7614)
  line L61 (-573, 222.7614) -> (-447, 222.7614)
  line L62 (-447, 241.7622) -> (-573, 241.7622)
  line L63 (-573, 306.7622) -> (-573, 241.7622)
  line L64 (-447, 306.7622) -> (-573, 306.7622)
  line L65 (-447, 306.7622) -> (-447, 241.7622)
  line L66 (-169.076, 354.2783) -> (-351.2252, 354.2783)
  line L67 (-169.076, 419.2783) -> (-169.076, 354.2783)
  line L68 (-351.2252, 419.2783) -> (-351.2252, 354.2783)
  line L69 (-351.2252, 419.2783) -> (-169.076, 419.2783)
  line L70 (-389.076, 354.2783) -> (-571.2252, 354.2783)
  line L71 (-389.076, 419.2783) -> (-389.076, 354.2783)
  line L72 (-571.2252, 419.2783) -> (-571.2252, 354.2783)
  line L73 (-571.2252, 419.2783) -> (-389.076, 419.2783)
sketch "Sketch24" plane through (0, -169.1114, 0) normal (0, -1, 0) x (1, 0, 0)
  line L0 (-63, -145.2447) -> (63, -145.2447)
  line L1 (63, -145.2447) -> (63, -80.2447)
  line L2 (63, -80.2447) -> (-63, -80.2447)
  line L3 (-63, -80.2447) -> (-63, -145.2447)
  line L4 (63, -73.8947) -> (-63, -73.8947)
  line L5 (-63, -80.2447) -> (-63, -145.2447)
  line L6 (-63, -145.2447) -> (-63, -151.5947)
  line L7 (63, -151.5947) -> (-63, -151.5947)
  line L8 (63, -80.2447) -> (63, -145.2447)
  line L9 (63, -145.2447) -> (63, -151.5947)
  line L10 (63, -80.2447) -> (63, -73.8947)
  line L11 (-63, -73.8947) -> (-63, -80.2447)
  point P0 (-63, -73.8947)
  point P1 (-63, -145.2447)
sketch "Sketch25" plane through (0, -38.3761, 22.1564) normal (0, -0.866025, 0.5) x (1, 0, 0)
  line L0 (50, 71.5294) -> (50, -88.4706)
  line L1 (50, -88.4706) -> (-50, -88.4706)
  line L2 (-50, -88.4706) -> (-50, 71.5294)
  line L3 (-50, 71.5294) -> (50, 71.5294)
  line L4 (63, 84.5294) -> (-63, 84.5294)
  line L5 (-63, 84.5294) -> (-63, -101.4706)
  line L6 (-63, -101.4706) -> (63, -101.4706)
  line L7 (63, -101.4706) -> (63, 84.5294)
  line L8 (-63, 82.9419) -> (63, 82.9419)
  line L9 (50, 71.5294) -> (-50, 71.5294)
  line L10 (-63, 84.5294) -> (-63, -101.4706)
  line L11 (-50, 71.5294) -> (-50, -88.4706)
  line L12 (50, -88.4706) -> (50, 71.5294)
  line L13 (63, 84.5294) -> (63, -101.4706)
  line L14 (-50, -88.4706) -> (50, -88.4706)
  line L15 (-63, -101.4706) -> (63, -101.4706)
extrude "Extrude41" cut 1 faces at (16.6667, -80.7783, -55.5197) along direction (0, -0.5, -0.866025) blind 2.5 on bodies 1 bodies 1 17
extrude "Extrude42" cut 1 faces at (16.6667, 1.0548, 81.986) along direction (0, 0.5, 0.866025) blind 2.5 on bodies 1 bodies 1 17
extrude "Extrude43" cut 1 faces at (-50, -52.6952, -11.1117) along direction (-1, 0, 0) blind 2 on bodies 17 bodies 1 17
extrude "Extrude44" cut 1 faces at (50, -54.5283, -10.0534) along direction (1, 0, 0) blind 2 on bodies 17 bodies 1 17
copy_body "CopyPasteBodies16" bodies 1 makes body 30
move_body "Move35" bodies 30 to x (1, 0, 0) y (0, 1, 0) z (0, 0, 1) at (-140, 0, 0)
move_body "Align18" bodies 30 to x (1, 0, 0) y (0, -0.5, 0.866025) z (0, -0.866025, -0.5) at (0, -45.5828, 37.9629)
sketch "Sketch26" plane through (0, 0, 0) normal (0, 0, 1) x (-1, 0, 0)
  line L0 (192, -45.3878) -> (88, -45.3878)
  line L1 (88, -45.3878) -> (88, 119.6122)
  line L2 (88, 119.6122) -> (192, 119.6122)
  line L3 (192, 119.6122) -> (192, -45.3878)
  line L4 (203, 130.1122) -> (77, 130.1122)
  line L5 (77, 130.1122) -> (77, -55.8878)
  line L6 (77, -55.8878) -> (203, -55.8878)
  line L7 (203, -55.8878) -> (203, 130.1122)
  line L8 (88, 119.6122) -> (88, -45.3878)
  line L9 (192, -45.3878) -> (192, 119.6122)
  line L10 (192, 119.6122) -> (88, 119.6122)
  line L11 (88, -45.3878) -> (192, -45.3878)
  line L12 (203, 130.1122) -> (203, -55.8878)
  line L13 (203, -55.8878) -> (77, -55.8878)
  line L14 (77, -55.8878) -> (77, 130.1122)
  line L15 (77, 130.1122) -> (203, 130.1122)
hidden bodies 18 19 20 21 22 23 24 25 26 27 28 29 30
equation "wood_thickness = 0.25 in"
equation "art_thickness = ( 1 / 8 ) * 1 in"
equation "d7 = wood_thickness"
equation "d9 = wood_thickness"
equation "d10 = wood_thickness"
equation "d11 = wood_thickness"
equation "d12 = wood_thickness"
equation "d48 = -wood_thickness"
equation "d53 = -wood_thickness"
equation "d57 = -wood_thickness"
equation "d61 = wood_thickness"
equation "d63 = wood_thickness + 10 mm"
equation "d64 = d63"
equation "d65 = d64"
equation "d66 = d64"
equation "d70 = -wood_thickness"
equation "d76 = wood_thickness"
equation "d78 = wood_thickness"
equation "d82 = wood_thickness"
equation "d84 = wood_thickness"
equation "d86 = 126 mm - wood_thickness"
equation "d94 = -wood_thickness"
equation "d96 = wood_thickness"